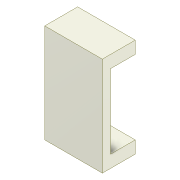
# Autodesk Inventor part: uchwyt_krancowka_alternatywa_2
Saved by Autodesk Inventor 2021 (Build 250183000, 183)
## iProperties
Created: 2022-09-08
Part Number: uchwyt_krancowka_alternatywa_2
Material: Generic
Document SubType Name: Modeling
Designer: agnpi
Density: 1 g/cm^3
Appearance: Smooth - Ivory
Author: agnpi
Autodesk Inventor part; units mm, degrees
ref_plane "YZ Plane" through (0, 0, 0) normal (1, 0, 0) x (0, 1, 0)
ref_plane "XZ Plane" through (0, 0, 0) normal (0, 1, 0) x (-1, 0, 0)
ref_plane "XY Plane" through (0, 0, 0) normal (0, 0, 1) x (1, 0, 0)
sketch "Sketch1" plane through (0, 0, 0) normal (0, 1, 0) x (-1, 0, 0)
  line L0 (9.8, 0) -> (-9.8, 0) projected
  line L1 (0, -5.6) -> (0, 5.6) projected
  line L2 (-7, 4) -> (7, 4)
  line L3 (7, 4) -> (7, -4)
  line L4 (7, -4) -> (-7, -4)
  line L5 (-7, -4) -> (-7, 4)
  line L6 (-7, 4) -> (7, -4) construction
  line L7 (7, 4) -> (-7, -4) construction
  point P0 (0, 0)
  dimension "d0" = 14
  dimension "d1" = 8
  constraints: 12 end point, 2 midpoint, 2 parallel, 1 horizontal, 1 perpendicular
  measures "d0" distance of L3.end L4.end
  measures "d1" distance of L2.end L3.end
extrude "Extrusion1" add sketch "Sketch1" along normal blind 3
sketch "Sketch2" plane through (0, 3, 0) normal (0, 1, 0) x (1, 0, 0)
  line L0 (-7, 4) -> (-7, -4) projected
  line L1 (7, -4) -> (7, 4) projected
  line L2 (-7, -4) -> (7, -4)
  line L3 (7, -4) -> (7, -2)
  line L4 (7, -2) -> (-7, -2)
  line L5 (-7, -2) -> (-7, -4)
  point P0 (0, 0)
  point P1 (-7, -2)
  dimension "d4" = 2
  constraints: 8 end point, 2 parallel, 1 horizontal, 1 perpendicular, 1 point on line
  measures "d4" distance between parallel lines of L2 L4
extrude "Extrusion2" add sketch "Sketch2" along normal blind 21
sketch "Sketch3" plane through (7, 3, 2) normal (0, 0, -1) x (-1, 0, 0)
  line L0 (0, -3) -> (0, 21) projected
  line L1 (14, -3) -> (14, 21) projected
  line L2 (0, 21) -> (14, 21)
  line L3 (14, 21) -> (14, 18)
  line L4 (14, 18) -> (0, 18)
  line L5 (0, 18) -> (0, 21)
  point P0 (7, -3)
  point P1 (0, 18)
  dimension "d7" = 3
  constraints: 8 end point, 2 parallel, 1 horizontal, 1 perpendicular, 1 point on line
  measures "d7" distance of L2.end L3.end
extrude "Extrusion3" add sketch "Sketch3" along normal up to surface (6 mm away)
body "Solid1"
